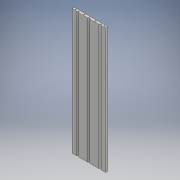
# Autodesk Inventor part: coverplate
Saved by Autodesk Inventor 2018 (Build 220112000, 112)
## iProperties
Created: 2018-06-04
Part Number: coverplate
Material: Generic
Document SubType Name: Modeling
Designer: John Viljoen
Density: 1 g/cm^3
Appearance: Default
Author: John Viljoen
Autodesk Inventor part; units mm, degrees
ref_plane "YZ Plane" through (0, 0, 0) normal (1, 0, 0) x (0, 1, 0)
ref_plane "XZ Plane" through (0, 0, 0) normal (0, 1, 0) x (-1, 0, 0)
ref_plane "XY Plane" through (0, 0, 0) normal (0, 0, 1) x (1, 0, 0)
sketch "Sketch1" plane through (0, 0, 0) normal (0, 0, 1) x (1, 0, 0)
  line L0 (0, 0) -> (0, 6.35)
  line L1 (0, 6.35) -> (97.04, 6.35)
  line L2 (97.04, 6.35) -> (97.04, 0)
  line L3 (97.04, 0) -> (0, 0)
  dimension "d0" = 6.35
  dimension "d1" = 97.04
  constraints: 8 end point, 2 perpendicular, 1 horizontal, 1 vertical
  measures "d0" distance of L0.start L0.end
  measures "d1" distance of L0.end L1.end
extrude "Extrusion1" add sketch "Sketch1" along normal blind 332
sketch "Sketch2" plane through (0, 0, 332) normal (0, 0, 1) x (1, 0, 0)
  line L0 (0, 0) -> (16.1733, 0) construction
  line L1 (16.1733, 0) -> (48.52, 0) construction
  line L2 (48.52, 0) -> (80.8667, 0) construction
  line L3 (0, 0) -> (97.04, 0) projected
  arc A0 (19.3483, 0) -> (12.9983, 0) centre (16.1733, 0) ccw
  arc A1 (51.695, 0) -> (45.345, 0) centre (48.52, 0) ccw
  arc A2 (84.0417, 0) -> (77.6917, 0) centre (80.8667, 0) ccw
  line L4 (12.9983, 0) -> (19.3483, 0)
  line L5 (45.345, 0) -> (51.695, 0)
  line L6 (77.6917, 0) -> (84.0417, 0)
  dimension "d4" = 16.1733
  dimension "d5" = 32.3467
  dimension "d6" = 32.3467
  dimension "d12" = 3.175
  dimension "d13" = 3.175
  dimension "d14" = 3.175
  constraints: 12 end point, 6 point on circle, 5 point on line, 3 centre point, 3 coincident, 3 collinear
  measures "d4" distance of L0.start L0.end
  measures "d5" distance of L0.end L1.end
  measures "d6" distance of L1.end L2.end
  measures "d12" radius of A0
  measures "d13" radius of A1
  measures "d14" radius of A2
extrude "Extrusion3" cut sketch "Sketch2" against normal through all
sketch "Sketch3" plane through (0, 0, 332) normal (0, 0, 1) x (1, 0, 0)
  arc A0 (19.3483, 0) -> (12.9983, 0) centre (16.1733, 0) ccw projected
  line L0 (0, 0) -> (0, 6.35) construction
  line L1 (0, 0) -> (0, 3.175) construction
  arc A1 (19.3483, 0) -> (12.9983, 0) centre (16.1733, 0) ccw construction
  line L2 (16.1733, 3.175) -> (12.9983, 3.175)
  line L3 (0, 3.175) -> (6.4992, 3.175) construction
  line L4 (45.345, 0) -> (19.3483, 0) construction
  line L5 (19.3483, 0) -> (32.3467, 0) construction
  circle A2 centre (32.3467, 3.175) radius 1.5
  circle A3 centre (6.4992, 3.175) radius 1.5
  line L6 (51.695, 0) -> (64.6933, 0) construction
  line L7 (77.6917, 0) -> (51.695, 0) construction
  circle A4 centre (64.6933, 3.175) radius 1.5
  line L8 (84.0417, 0) -> (90.5408, 0) construction
  line L9 (97.04, 0) -> (84.0417, 0) construction
  circle A5 centre (90.5408, 3.175) radius 1.5
  dimension "d17" = 3
  dimension "d18" = 3
  dimension "d19" = 3
  dimension "d20" = 3
  constraints: 12 end point, 4 centre point, 4 midpoint, 2 horizontal, 2 point on circle, 2 tangent, 1 coincident
  measures "d17" diameter of A2
  measures "d18" diameter of A3
  measures "d19" diameter of A4
  measures "d20" diameter of A5
extrude "Extrusion4" cut sketch "Sketch3" against normal blind 20
sketch "Sketch4" plane through (0, 0, 0) normal (0, 0, -1) x (-1, 0, 0)
  circle A0 centre (-6.4992, 3.175) radius 1.5
  circle A1 centre (-32.3467, 3.175) radius 1.5
  circle A2 centre (-64.6933, 3.175) radius 1.5
  circle A3 centre (-90.5408, 3.175) radius 1.5
  dimension "d23" = 3
  dimension "d24" = 3
  dimension "d25" = 3
  dimension "d26" = 3
  constraints: 4 centre point
  measures "d23" diameter of A0
  measures "d24" diameter of A1
  measures "d25" diameter of A2
  measures "d26" diameter of A3
extrude "Extrusion5" cut sketch "Sketch4" against normal blind 20
sketch "Sketch5" plane through (0, 0, 332) normal (0, 0, 1) x (1, 0, 0)
  circle A0 centre (64.6933, 3.175) radius 1.5 projected
  circle A1 centre (32.3467, 3.175) radius 1.5 projected
  circle A2 centre (6.4992, 3.175) radius 1.5 projected
  circle A3 centre (90.5408, 3.175) radius 1.5 projected
  arc A4 (51.695, 0) -> (45.345, 0) centre (48.52, 0) ccw projected
  line L0 (51.695, 0) -> (77.6917, 0) projected
  arc A5 (84.0417, 0) -> (77.6917, 0) centre (80.8667, 0) ccw projected
  line L1 (84.0417, 0) -> (97.04, 0) projected
  line L2 (97.04, 0) -> (97.04, 6.35) projected
  line L3 (97.04, 6.35) -> (0, 6.35) projected
  line L4 (0, 6.35) -> (0, 0) projected
  line L5 (0, 0) -> (12.9983, 0) projected
  arc A6 (19.3483, 0) -> (12.9983, 0) centre (16.1733, 0) ccw projected
  line L6 (19.3483, 0) -> (45.345, 0) projected
extrude "Extrusion6" add sketch "Sketch5" along normal blind 30.87
body "Solid1"
